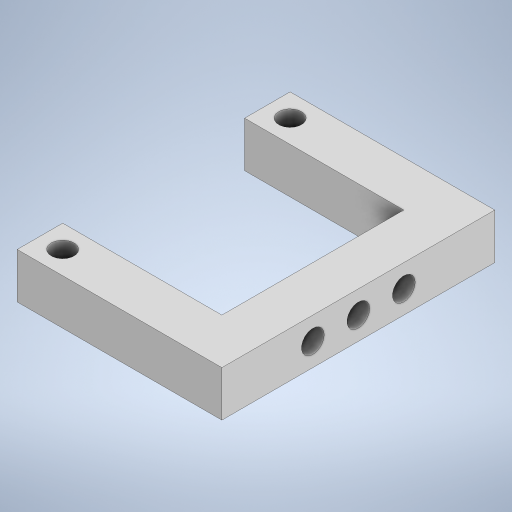
# Autodesk Inventor part: Скоба для полки
Saved by Autodesk Inventor 2023 (Build 270158000, 158)
## iProperties
Created: 2022-05-19
Part Number: Скоба для полки
Material: Типовые
Document SubType Name: Modeling
Designer: avkap
Density: 1 g/cm^3
Appearance: По умолчанию
Author: avkap
Autodesk Inventor part; units mm, degrees
ref_plane "YZ Plane" through (0, 0, 0) normal (1, 0, 0) x (0, 1, 0)
ref_plane "XZ Plane" through (0, 0, 0) normal (0, 1, 0) x (-1, 0, 0)
ref_plane "XY Plane" through (0, 0, 0) normal (0, 0, 1) x (1, 0, 0)
sketch "Эскиз1" plane through (0, 0, 0) normal (0, 1, 0) x (-1, 0, 0)
  line L0 (0, 0) -> (90, 0)
  line L1 (90, 0) -> (90, -20)
  line L2 (90, -20) -> (20, -20)
  line L3 (0, 0) -> (0, -120)
  line L4 (0, -120) -> (90, -120)
  line L5 (90, -120) -> (90, -100)
  line L6 (90, -100) -> (20, -100)
  line L7 (20, -100) -> (20, -20)
  line L8 (90, 0) -> (90, -10)
  line L9 (90, -10) -> (80, -10)
  line L10 (90, -100) -> (90, -110)
  line L11 (90, -110) -> (80, -110)
  circle A0 centre (80, -10) radius 5
  circle A1 centre (80, -110) radius 5
  dimension "d4" = 90
  dimension "d5" = 20
  dimension "d6" = 70
  dimension "d7" = 120
  dimension "d8" = 20
  dimension "d9" = 10
  dimension "d10" = 10
  dimension "d11" = 10
  dimension "d12" = 10
  dimension "d13" = 10
  dimension "d14" = 10
  constraints: 24 end point, 8 perpendicular, 2 centre point, 2 coincident, 2 midpoint, 2 point on line, 1 horizontal
  measures "d4" distance of L0.start L0.end
  measures "d5" distance of L0.end L1.end
  measures "d6" distance of L1.end L2.end
  measures "d7" distance of L0.start L3.end
  measures "d8" distance of L4.end L5.end
  measures "d9" distance of L0.end L8.end
  measures "d10" distance of L8.end L9.end
  measures "d11" distance of L5.end L10.end
  measures "d12" distance of L10.end L11.end
  measures "d13" diameter of A0
  measures "d14" diameter of A1
extrude "Выдавливание1" add sketch "Эскиз1" along normal blind 20
sketch "Эскиз2" plane through (-20, 0, -100) normal (-1, 0, 0) x (0, 0, 1)
  line L0 (80, 0) -> (80, 20) projected
  line L1 (80, 0) -> (80, 10)
  line L2 (80, 10) -> (0, 10)
  line L3 (0, 0) -> (0, 20) projected
  circle A0 centre (40, 10) radius 5
  line L4 (40, 10) -> (60, 10)
  circle A1 centre (60, 10) radius 5
  line L5 (40, 10) -> (20, 10)
  circle A2 centre (20, 10) radius 5
  point P0 (100, 0)
  dimension "d17" = 10
  dimension "d18" = 20
  dimension "d19" = 10
  dimension "d20" = 20
  dimension "d21" = 10
  constraints: 8 end point, 3 centre point, 3 midpoint, 2 coincident, 2 point on line
  measures "d17" diameter of A0
  measures "d18" distance of L4.start L4.end
  measures "d19" diameter of A1
  measures "d20" distance of L4.start L5.end
  measures "d21" diameter of A2
extrude "Выдавливание2" cut sketch "Эскиз2" against normal blind 95.75
